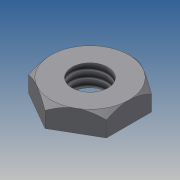
# Autodesk Inventor part: Mutter_ra8846s
Saved by Autodesk Inventor 2021 (Build 250183000, 183)
## iProperties
Created: 2020-12-18
Part Number: Mutter_ra8846s
Material: Allgemein
Document SubType Name: Modeling
Designer: Sander
Density: 1 g/cm^3
Appearance: Vorgabe
Author: Sander
Autodesk Inventor part; units mm, degrees
ref_plane "YZ-Ebene" through (0, 0, 0) normal (1, 0, 0) x (0, 1, 0)
ref_plane "XZ-Ebene" through (0, 0, 0) normal (0, 1, 0) x (-1, 0, 0)
ref_plane "XY-Ebene" through (0, 0, 0) normal (0, 0, 1) x (1, 0, 0)
sketch "Skizze1" plane through (0, 0, 0) normal (0, 0, 1) x (1, 0, 0)
  line L0 (-3.78, 0) -> (3.78, 0) projected
  line L1 (0, -4.3648) -> (0, 4.3648) projected
  line L2 (0, 3.1177) -> (2.7, 1.5588)
  line L3 (2.7, 1.5588) -> (2.7, -1.5588)
  line L4 (2.7, -1.5588) -> (0, -3.1177)
  line L5 (0, -3.1177) -> (-2.7, -1.5588)
  line L6 (-2.7, -1.5588) -> (-2.7, 1.5588)
  line L7 (-2.7, 1.5588) -> (0, 3.1177)
  point P0 (0, 0)
  point P1 (0, 0)
  dimension "d0" = 5.4
  constraints: 12 end point, 1 coincident, 1 point on line, 13 other
  measures "d0" distance between parallel lines of L3 L6
extrude "Extrusion1" add sketch "Skizze1" along normal blind 1.6
sketch "Skizze2" plane through (0, 0, 1.6) normal (0, 0, 1) x (1, 0, 0)
  line L0 (0, 3.1177) -> (-2.7, 1.5588) projected
  circle A0 centre (0, 0) radius 2.7
  constraints: 1 centre point, 1 coincident, 1 tangent
extrude "Extrusion2" cut sketch "Skizze2" against normal blind 1.5 draft 45 keep common part
sketch "Skizze3" plane through (0, 0, 1.6) normal (0, 0, 1) x (1, 0, 0)
  arc A0 (-2.7, 0) -> (-1.35, -2.3383) centre (0, 0) ccw projected
  circle A1 centre (0, 0) radius 1.25
  dimension "d5" = 2.5
  constraints: 1 centre point, 1 coincident
  measures "d5" diameter of A1
extrude "Extrusion3" cut sketch "Skizze3" against normal blind 1.5
thread "Gewinde1" size "M3x0.5" class "6H" standard "ANSI Metric M Profile" length 7
